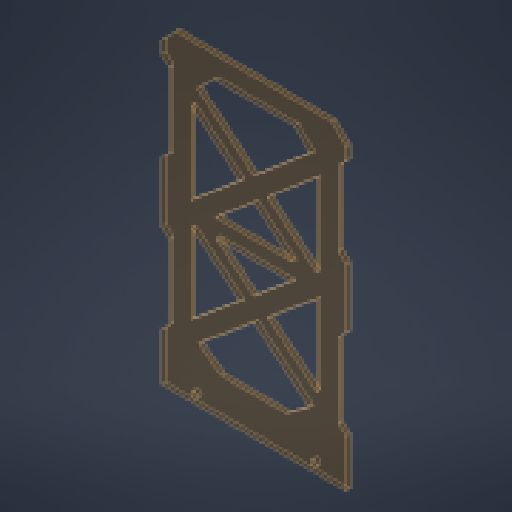
# Autodesk Inventor part: Shelf2
Saved by Autodesk Inventor 2023.4 (Build 274418000, 418)
## iProperties
Created: 2025-10-22
Part Number: Shelf2
Material: Generic
Document SubType Name: Modeling
Designer: Malthe Sennels
Density: 1 g/cm^3
Appearance: Polycarbonate - Smoked
Author: Malthe Sennels
Autodesk Inventor part; units mm, degrees
ref_plane "YZ Plane" through (0, 0, 0) normal (1, 0, 0) x (0, 1, 0)
ref_plane "XZ Plane" through (0, 0, 0) normal (0, 1, 0) x (-1, 0, 0)
ref_plane "XY Plane" through (0, 0, 0) normal (0, 0, 1) x (1, 0, 0)
sketch "Sketch1" plane through (0, 0, 0) normal (0, 0, 1) x (1, 0, 0)
  line L0 (0, 0) -> (-124, 0)
  line L1 (-124, 0) -> (-124, 210)
  line L2 (-124, 210) -> (0, 210)
  line L3 (0, 210) -> (0, 0)
  circle A0 centre (-22, 5) radius 2.25 projected
  circle A1 centre (-102, 5) radius 2.25 projected
  dimension "d0" = 124
  dimension "d1" = 210
  constraints: 8 end point, 2 parallel, 1 horizontal, 1 perpendicular
  measures "d0" distance of L1.end L2.end
  measures "d1" distance of L0.end L1.end
extrude "Extrusion1" add sketch "Sketch1" along normal blind 3
sketch "Sketch2" plane through (0, 0, 0) normal (0, 0, -1) x (-1, 0, 0)
  line L0 (84, 25) -> (40, 25) projected
  line L1 (99.0611, 36.2959) -> (84, 25) projected
  line L2 (62, 66.8593) -> (99.0611, 36.2959) projected
  line L3 (24.9389, 36.2959) -> (62, 66.8593) projected
  line L4 (40, 25) -> (24.9389, 36.2959) projected
  line L5 (52.5695, 74.6364) -> (20, 47.7771) projected
  line L6 (20, 101.4957) -> (52.5695, 74.6364) projected
  line L7 (20, 47.7771) -> (20, 101.4957) projected
  line L8 (62, 82.4135) -> (36.7061, 103.2728) projected
  line L9 (62, 152.48) -> (24.2582, 184.2582) projected
  line L10 (99.7418, 184.2582) -> (62, 152.48) projected
  line L11 (35, 195) -> (89, 195) projected
  line L12 (89, 195) -> (99.7418, 184.2582) projected
  line L13 (24.2582, 184.2582) -> (35, 195) projected
  line L14 (20, 117.1164) -> (20, 172.1564) projected
  line L15 (20, 172.1564) -> (52.6844, 144.6364) projected
  line L16 (52.6844, 144.6364) -> (20, 117.1164) projected
  line L17 (104, 117.1164) -> (71.3156, 144.6364) projected
  line L18 (71.3156, 144.6364) -> (104, 172.1564) projected
  line L19 (104, 172.1564) -> (104, 117.1164) projected
  line L20 (71.4305, 74.6364) -> (104, 101.4957) projected
  line L21 (104, 101.4957) -> (104, 47.7771) projected
  line L22 (104, 47.7771) -> (71.4305, 74.6364) projected
  line L23 (87.2939, 103.2728) -> (62, 82.4135) projected
  line L24 (36.7061, 103.2728) -> (87.2939, 103.2728) projected
  line L25 (87.5585, 115.2728) -> (36.4415, 115.2728) projected
  line L26 (62, 136.7928) -> (87.5585, 115.2728) projected
  line L27 (36.4415, 115.2728) -> (62, 136.7928) projected
  line L28 (119, 137) -> (119, 187) projected
  line L29 (119, 187) -> (124, 192) projected
  line L30 (124, 200.3422) -> (114.3422, 210) projected
  line L31 (9.6578, 210) -> (0, 200.3422) projected
  line L32 (0, 192) -> (5, 187) projected
  line L33 (5, 187) -> (5, 137) projected
  line L34 (5, 137) -> (0, 132) projected
  line L35 (0, 92) -> (5, 87) projected
  line L36 (5, 87) -> (5, 37) projected
  line L37 (5, 37) -> (0, 32) projected
  line L38 (124, 132) -> (119, 137) projected
  line L39 (119, 87) -> (124, 92) projected
  line L40 (119, 37) -> (119, 87) projected
  line L41 (124, 32) -> (119, 37) projected
  line L42 (0, 210) -> (124, 210) projected
  line L43 (0, 0) -> (124, 0)
  line L44 (124, 0) -> (124, 210)
  line L45 (124, 210) -> (0, 210)
  line L46 (0, 210) -> (0, 0)
  constraints: 8 end point, 2 parallel, 1 horizontal, 1 perpendicular
extrude "Extrusion2" cut sketch "Sketch2" against normal through all contours L0 L4 L3 L2 L1 | L5 L7 L6 | L8 L24 L23 | L9 L13 L11 L12 L10 | L14 L15 L16 | L17 L18 L19 | L20 L21 L22 | L25 L27 L26 | L28 L29 L44 L38 | L44 L41 L40 L39 | L30 L42 L44 | L31 L46 L42 | L46 L35 L36 L37 | L32 L33 L34 L46
ref_plane "Work Plane1" through (20, 112, 3) normal (0, -1, 0) x (0, 0, -1)
body "Solid1"
